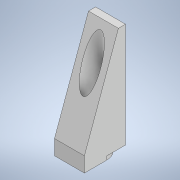
# Autodesk Inventor part: rpi_stand
Saved by Autodesk Inventor 2020 (Build 240168000, 168)
## iProperties
Created: 2020-12-18
Part Number: rpi_stand
Material: Generic
Document SubType Name: Modeling
Designer: agupta40
Density: 1 g/cm^3
Appearance: Default
Author: agupta40
Autodesk Inventor part; units mm, degrees
ref_plane "YZ Plane" through (0, 0, 0) normal (1, 0, 0) x (0, 1, 0)
ref_plane "XZ Plane" through (0, 0, 0) normal (0, 1, 0) x (-1, 0, 0)
ref_plane "XY Plane" through (0, 0, 0) normal (0, 0, 1) x (1, 0, 0)
sketch "Sketch1" plane through (0, 0, 0) normal (1, 0, 0) x (0, 1, 0)
  line L0 (0, 0) -> (0, 11)
  line L1 (0, 11) -> (3, 11)
  line L2 (3, 11) -> (28, 1.9007)
  line L3 (28, 1.9007) -> (28, 0)
  line L4 (28, 0) -> (0, 0)
  dimension "d0" = 11
  dimension "d1" = 160
  dimension "d2" = 25
  dimension "d4" = 3
  constraints: 10 end point, 2 perpendicular, 1 parallel, 1 vertical
  measures "d0" distance of L0.start L0.end
  measures "d1" angle of L1 L2
  measures "d2" horizontal distance of L1.end L2.end
  measures "d4" distance of L0.end L1.end
extrude "Extrusion1" add sketch "Sketch1" along normal blind 8
sketch "Sketch2" plane through (0, 0, 0) normal (0, -1, 0) x (1, 0, 0)
  circle A0 centre (4, 5) radius 4
  line L0 (0, 11) -> (0, 0) projected
  line L1 (8, 11) -> (8, 0) projected
  line L2 (0, 0) -> (8, 0) projected
  circle A1 centre (4, 5) radius 3.125
  circle A2 centre (4, 5) radius 1.375
  line L3 (0, 11) -> (8, 11) projected
  dimension "d7" = 6.25
  dimension "d8" = 2.75
  dimension "d20" = 6
  constraints: 3 centre point, 2 coincident, 2 tangent
  measures "d7" diameter of A1
  measures "d8" diameter of A2
  measures "d20" distance from line of L3 A0.centre
extrude "Extrusion2" cut sketch "Sketch2" against normal through all contours A2
extrude "Extrusion3" cut sketch "Sketch2" against normal blind 4.25 contours A1
extrude "Extrusion4" add sketch "Sketch2" along normal blind 1 contours A0
sketch "Sketch3" plane through (0, 28, 1.9007) normal (0, 1, 0) x (1, 0, 0)
  circle A0 centre (4, -3.0993) radius 2.375
  circle A1 centre (4, -3.0993) radius 1.375 projected
  point P0 (0, 1.9007)
  point P1 (4, -1.5531)
  dimension "d15" = 4.75
  constraints: 1 centre point, 1 concentric
  measures "d15" diameter of A0
extrude "Extrusion5" cut sketch "Sketch3" against normal blind 22.75 contours A0 | A1
sketch "Sketch4" plane through (0, 0, 11) normal (0, -1, 0) x (1, 0, 0)
  arc A0 (8, -6) -> (0, -6) centre (4, -6) ccw projected
  line L0 (8, 0) -> (8, -6) projected
  line L1 (0, 0) -> (8, 0) projected
  line L2 (0, 0) -> (0, -6) projected
  point P0 (0, -11)
extrude "Extrusion6" add sketch "Sketch4" along normal up to surface (1 mm away)
body "Solid1"
